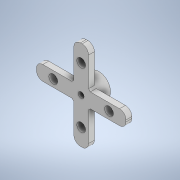
# Autodesk Inventor part: ServoESP32V3Arm
Saved by Autodesk Inventor 2020 (Build 240168000, 168)
## iProperties
Created: 2022-11-25
Part Number: ServoESP32V3Arm
Material: Generic
Document SubType Name: Modeling
Designer: agraa4529
Density: 1 g/cm^3
Appearance: Default
Author: agraa4529
## iProperties of the stored document _3DPrint.ipt
Created: 2022-11-29
Part Number: _3DPrint
Material: Generic
Document SubType Name: Modeling
Designer: agraa4529
Density: 1 g/cm^3
Appearance: Default
Author: agraa4529
Autodesk Inventor part; units mm, degrees
ref_plane "YZ Plane" through (0, 0, 0) normal (1, 0, 0) x (0, 1, 0)
ref_plane "XZ Plane" through (0, 0, 0) normal (0, 1, 0) x (-1, 0, 0)
ref_plane "XY Plane" through (0, 0, 0) normal (0, 0, 1) x (1, 0, 0)
sketch "Sketch2" plane through (0, 0, 0) normal (0, 0, 1) x (1, 0, 0)
  circle A0 centre (0, 0) radius 4
  circle A1 centre (0, 0) radius 2.5
  dimension "d7" = 8
  dimension "d36" = 5
  constraints: 2 centre point, 2 coincident
  measures "d7" diameter of A0
  measures "d36" diameter of A1
extrude "Extrusion1" add sketch "Sketch2" along normal blind 4
sketch "Sketch3" plane through (0, 0, 4) normal (0, 0, 1) x (1, 0, 0)
  circle A0 centre (0, 0) radius 1
  circle A1 centre (0, 0) radius 4
  dimension "d16" = 2
  constraints: 2 centre point, 2 coincident
  measures "d16" diameter of A0
extrude "Extrusion2" add sketch "Sketch3" along normal blind 2
sketch "Sketch4" plane through (0, 0, 6) normal (0, 0, 1) x (1, 0, 0)
  circle A0 centre (0, 0) radius 4 projected
  line L0 (-2.5, 15.2615) -> (2.5, 15.2615)
  line L1 (2.5, 15.2615) -> (2.5, 3.7385)
  line L2 (-2.5, 3.7385) -> (-2.5, 15.2615)
  line L3 (-2.5, 15.2615) -> (2.5, 3.7385) construction
  line L4 (2.5, 15.2615) -> (-2.5, 3.7385) construction
  line L5 (2.5, 3.7385) -> (2.5, 3.1225)
  line L6 (2.5, 3.1225) -> (-2.5, 3.1225)
  line L7 (-2.5, 3.1225) -> (-2.5, 3.7385)
  line L8 (-3.7385, -2.5) -> (-15.2615, -2.5)
  line L9 (-15.2615, -2.5) -> (-15.2615, 2.5)
  line L10 (-15.2615, 2.5) -> (-3.7385, 2.5)
  line L11 (-3.1225, 2.5) -> (-3.1225, -2.5)
  line L12 (-3.1225, -2.5) -> (-3.7385, -2.5)
  line L13 (-3.7385, 2.5) -> (-3.1225, 2.5)
  line L14 (2.5, -3.7385) -> (2.5, -15.2615)
  line L15 (2.5, -15.2615) -> (-2.5, -15.2615)
  line L16 (-2.5, -15.2615) -> (-2.5, -3.7385)
  line L17 (-2.5, -3.1225) -> (2.5, -3.1225)
  line L18 (2.5, -3.1225) -> (2.5, -3.7385)
  line L19 (-2.5, -3.7385) -> (-2.5, -3.1225)
  line L20 (3.7385, 2.5) -> (15.2615, 2.5)
  line L21 (15.2615, 2.5) -> (15.2615, -2.5)
  line L22 (15.2615, -2.5) -> (3.7385, -2.5)
  line L23 (3.1225, -2.5) -> (3.1225, 2.5)
  line L24 (3.1225, 2.5) -> (3.7385, 2.5)
  line L25 (3.7385, -2.5) -> (3.1225, -2.5)
  circle A1 centre (9.5, 0) radius 1.5
  circle A2 centre (0, 9.5) radius 1.5
  circle A3 centre (-9.5, 0) radius 1.5
  circle A4 centre (0, -9.5) radius 1.5
  point P0 (0, 9.5)
  point P1 (-3.1225, -2.5)
  dimension "d20" = 5
  dimension "d21" = 11.523
  dimension "d22" = 0.616
  dimension "d23" = 5
  dimension "d26" = 360
  dimension "d31" = 3
  dimension "d34" = 360
  constraints: 52 end point, 4 centre point, 2 midpoint, 2 parallel, 1 horizontal, 1 perpendicular, 64 other
  measures "d20" distance of L1.end L2.start
  measures "d21" distance of L0.end L1.end
  measures "d22" distance of L5.start L5.end
  measures "d23" distance of L0.start L0.end
  measures "d31" diameter of A1
extrude "Extrusion3" add sketch "Sketch4" against normal blind 2 contours A0 L24 L20 L21 L22 L25 | A0 L7 L2 L0 L1 L5 | L18 L14 L15 L16 L19 A0 | A0 L12 L8 L9 L10 L13
fillet "Fillet1" radius 2.2 8 edges at (2.5, -15.2615, 5) (-15.2615, -2.5, 5) (-15.2615, 2.5, 5) (-2.5, 15.2615, 5) (2.5, 15.2615, 5) (15.2615, 2.5, 5) (15.2615, -2.5, 5) (-2.5, -15.2615, 5)
body "Solid1"
